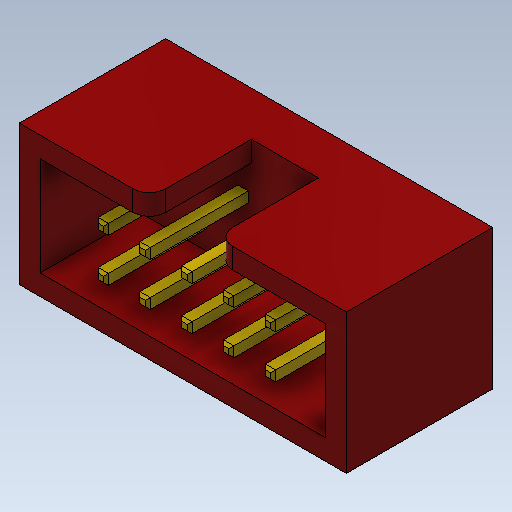
# Autodesk Inventor part: RC Male Connector
Saved by Autodesk Inventor 2020.1 (Build 241239000, 239)
## iProperties
Created: 2005-12-05
Part Number: RC Male Connector
Document SubType Name: Modeling
Designer: Simon.Ng@autodesk.com
Density: 1 g/cm^3
Mass: 0.847102 g
Surface Area: 12.4518 cm^2
Volume: 0.847102 cm^3
Material: Generic
Appearance: Red
Company: Autodesk Asia Pte. Ltd.
Title: PC Demo
Author: Simon.Ng@autodesk.com
Autodesk Inventor part; units mm, degrees
ref_plane "YZ Plane" through (0, 0, 0) normal (1, 0, 0) x (0, 1, 0)
ref_plane "XZ Plane" through (0, 0, 0) normal (0, 1, 0) x (-1, 0, 0)
ref_plane "XY Plane" through (0, 0, 0) normal (0, 0, 1) x (1, 0, 0)
sketch "Sketch1" plane through (0, 0, 0) normal (0, 0, 1) x (1, 0, 0)
  line L0 (0, 5.943) -> (0, -5.943) projected
  line L1 (-13.909, 0) -> (13.909, 0) projected
  line L2 (-9.935, 4.245) -> (9.935, 4.245)
  line L3 (9.935, 4.245) -> (9.935, -4.245)
  line L4 (9.935, -4.245) -> (-9.935, -4.245)
  line L5 (-9.935, -4.245) -> (-9.935, 4.245)
  dimension "d0" = 19.87
  dimension "d1" = 8.49
  constraints: 8 end point, 2 parallel, 1 horizontal, 1 perpendicular, 2 other
  measures "d0" distance of L2.start L2.end
  measures "d1" distance of L4.end L2.start
extrude "Extrusion1" add sketch "Sketch1" along normal blind 8.89
shell "Shell1" thickness 0.4 removed faces 1 at (-3.3117, 1.415, 8.89) ; own thickness 2.69 on faces at (-3.3117, 1.415, 0) ; own thickness 1.27 on faces at (9.935, 1.415, 2.9633) (-9.935, -1.415, 2.9633) ; own thickness 1.245 on faces at (3.3117, -4.245, 2.9633) (-3.3117, 4.245, 2.9633)
sketch "Sketch3" plane through (-9.935, 4.245, 0) normal (0, 1, 0) x (1, 0, 0)
  line L0 (0, -8.89) -> (19.87, -8.89) projected
  line L1 (9.935, 1.778) -> (9.935, -10.668) projected
  line L2 (7.903, -8.89) -> (11.967, -8.89)
  line L3 (11.967, -8.89) -> (11.967, -2.69)
  line L4 (7.903, -2.69) -> (7.903, -8.89)
  line L5 (11.967, -2.69) -> (7.903, -2.69)
  dimension "d10" = 4.064
  dimension "d31" = 6.2
  constraints: 8 end point, 2 perpendicular, 1 horizontal, 1 parallel, 1 point on line, 1 other
  measures "d10" distance of L2.start L2.end
  measures "d31" distance of L2.end L3.end
extrude "Extrusion3" cut sketch "Sketch3" against normal blind 1.778
sketch "Sketch4" plane through (-8.665, 3, 2.69) normal (0, 0, 1) x (1, 0, 0)
  line L0 (13.43, -1.57) -> (14.06, -1.57)
  line L1 (14.06, -1.57) -> (14.06, -2.2)
  line L2 (14.06, -2.2) -> (13.43, -2.2)
  line L3 (13.43, -2.2) -> (13.43, -1.57)
  line L4 (13.43, -4.2) -> (14.06, -4.2)
  line L5 (14.06, -4.2) -> (14.06, -4.83)
  line L6 (14.06, -4.83) -> (13.43, -4.83)
  line L7 (13.43, -4.83) -> (13.43, -4.2)
  line L8 (17.33, -6) -> (0, -6) projected
  line L9 (8.665, -6) -> (8.665, 1.245)
  line L10 (13.745, -2.2) -> (13.745, -4.2) construction
  line L11 (6.633, 1.245) -> (10.697, 1.245) projected
  dimension "d18" = 0.63
  dimension "d32" = 10.16
  constraints: 20 end point, 4 midpoint, 4 parallel, 3 perpendicular, 2 collinear, 2 horizontal
  measures "d18" distance of L0.start L0.end
  measures "d32" diameter of L10 L9
extrude "Extrusion4" add sketch "Sketch4" along normal blind 6.1
chamfer "Chamfer1" distance 0.15 angle 45 8 edges at (5.08, 0.8, 8.79) (4.765, 1.115, 8.79) (5.08, 1.43, 8.79) (5.395, 1.115, 8.79) (5.395, -1.515, 8.79) (5.08, -1.2, 8.79) (4.765, -1.515, 8.79) (5.08, -1.83, 8.79)
pattern_linear "Rectangular Pattern2" count 5 spacing 2.54 along (-1, 0, 0) of "Extrusion4", "Chamfer1"
fillet "Fillet1" radius 1 2 edges at (2.032, 3.6225, 8.89) (-2.032, 3.6225, 8.89)
body "Solid1"
